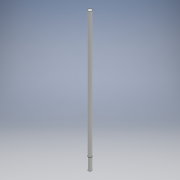
# Autodesk Inventor part: SMC_CJ2B16-175(円柱)
Saved by Autodesk Inventor 2018 (Build 220112000, 112)
## iProperties
Created: 2018-04-28
Part Number: SMC_CJ2B16-175(円柱)
Material: 一般
Document SubType Name: Modeling
Designer: Take
Density: 1 g/cm^3
Appearance: 既定
Author: Take
Autodesk Inventor part; units mm, degrees
ref_plane "YZ Plane" through (0, 0, 0) normal (1, 0, 0) x (0, 1, 0)
ref_plane "XZ Plane" through (0, 0, 0) normal (0, 1, 0) x (-1, 0, 0)
ref_plane "XY Plane" through (0, 0, 0) normal (0, 0, 1) x (1, 0, 0)
sketch "スケッチ1" plane through (0, 0, 0) normal (0, 1, 0) x (-1, 0, 0)
  line L0 (0, 0) -> (2.5, 0)
  line L1 (2.5, 0) -> (2.5, -182.5)
  line L2 (2.5, -182.5) -> (2.25, -183)
  line L3 (2.25, -183) -> (2.25, -200)
  line L4 (2.25, -200) -> (0, -200)
  line L5 (0, -200) -> (0, 0)
  point P0 (2.25, -182.5)
  dimension "d0" = 2.5
  dimension "d1" = 182.5
  dimension "d2" = 0.25
  dimension "d3" = 0.5
  dimension "d4" = 17
  constraints: 12 end point, 3 perpendicular, 1 horizontal, 1 vertical
  measures "d0" distance of L0.start L0.end
  measures "d1" distance of L0.end L1.end
  measures "d2" distance of L1.end point (2.25, -182.5)
  measures "d3" distance of L2.end point (2.25, -182.5)
  measures "d4" distance of L2.end L3.end
revolve "回転1" add sketch "スケッチ1" angle 360 about axis through (0, 0, -200) along (0, 0, 1)
